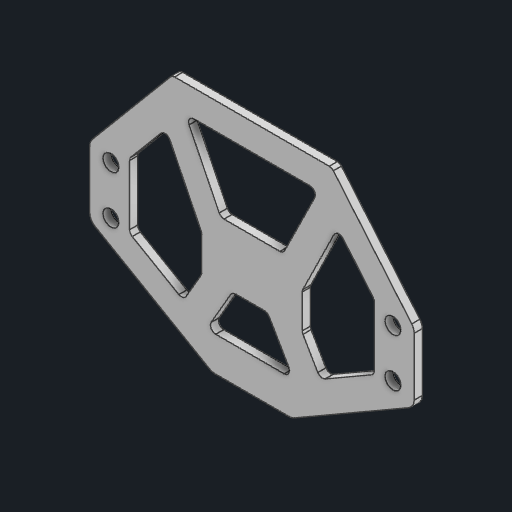
# Autodesk Inventor part: JawMount
Saved by Autodesk Inventor 2025.2 (Build 292293000, 293)
## iProperties
Created: 2024-12-21
Part Number: JawMount
Material: Generic
Document SubType Name: Sheet Metal
Designer: valer
Density: 1 g/cm^3
Sheet Metal Rule: Default
Appearance: Default
Author: valer
Autodesk Inventor part; units mm, degrees
ref_plane "YZ Plane" through (0, 0, 0) normal (1, 0, 0) x (0, 1, 0)
ref_plane "XZ Plane" through (0, 0, 0) normal (0, 1, 0) x (-1, 0, 0)
ref_plane "XY Plane" through (0, 0, 0) normal (0, 0, 1) x (1, 0, 0)
sketch "Sketch1" plane through (0, 0, 0) normal (0, 0, 1) x (1, 0, 0)
  circle A0 centre (-3.2439, -112.6362) radius 2.7 construction
  circle A1 centre (-3.2439, -130.6362) radius 2.7 construction
  line L0 (49.7615, -342.4426) -> (49.7615, 314.6303) construction
  line L1 (-11.2439, -109.7245) -> (-11.2439, -135.255)
  line L2 (-11.2439, -109.7245) -> (19.7615, -72.7737)
  line L3 (19.7615, -72.7737) -> (49.7615, -72.7737)
  circle A2 centre (-3.2439, -112.6362) radius 3
  circle A3 centre (-3.2439, -130.6362) radius 3
  line L4 (-11.2439, -135.255) -> (34.7615, -161.8162)
  line L5 (34.7615, -161.8162) -> (49.7615, -161.8162)
  line L6 (110.7669, -109.7245) -> (110.7669, -135.255)
  line L7 (110.7669, -109.7245) -> (79.7615, -72.7737)
  line L8 (79.7615, -72.7737) -> (49.7615, -72.7737)
  circle A4 centre (102.7669, -112.6362) radius 3
  circle A5 centre (102.7669, -130.6362) radius 3
  line L9 (110.7669, -135.255) -> (64.7615, -161.8162)
  line L10 (64.7615, -161.8162) -> (49.7615, -161.8162)
  point P0 (0, 0)
  dimension "d0" = 6
  dimension "d1" = 6
  dimension "d8" = 8
  dimension "d16" = 30
  dimension "d17" = 15
  dimension "d18" = 60
  dimension "d19" = 40
  dimension "d20" = 8
  dimension "d21" = 8
  measures "d0" diameter of A2
  measures "d1" diameter of A3
  measures "d8" distance from line of L2 A0.centre
  measures "d16" distance of L2.end L3.end
  measures "d17" distance of L4.end L5.end
  measures "d18" angle of L0 L4
  measures "d19" angle of L0 L2
  measures "d20" distance from line of A1.centre L1
  measures "d21" distance from line of L4 A3.centre
extrude "Plate1" add sketch "Sketch1" along normal blind 3.048
fillet "Fillet1" radius 4 6 edges at (-11.2439, -135.255, 1.524) (-11.2439, -109.7245, 1.524) (110.7669, -109.7245, 1.524) (110.7669, -135.255, 1.524) (64.7615, -161.8162, 1.524) (34.7615, -161.8162, 1.524)
sketch "Sketch2" plane through (0, 0, 3.048) normal (0, 0, 1) x (1, 0, 0)
  arc A0 (19.774, -118.0434) -> (18.9211, -121.2485) centre (16.9316, -119.0031) ccw projected
  arc A1 (80.0915, -120.6614) -> (80.0915, -117.3448) centre (82.5915, -119.0031) ccw projected
  arc A2 (47.082, -94.8758) -> (52.441, -94.8758) centre (49.7615, -96.225) ccw projected
  line L0 (3.7561, -107.7275) -> (3.7561, -132.1292)
  line L1 (3.7561, -107.7275) -> (17.5274, -91.3156)
  line L2 (17.5274, -91.3156) -> (30.8475, -118.3156)
  line L3 (30.8475, -118.3156) -> (30.8475, -131.9856)
  line L4 (30.8475, -131.9856) -> (24.0125, -143.8242)
  line L5 (24.0125, -143.8242) -> (3.7561, -132.1292)
  line L6 (24.6949, -82.7737) -> (38.0151, -109.7737)
  line L7 (38.0151, -109.7737) -> (61.508, -109.7737)
  line L8 (19.7615, -72.7737) -> (79.7615, -72.7737) projected
  line L9 (61.508, -109.7737) -> (74.8281, -82.7737)
  line L10 (74.8281, -82.7737) -> (24.6949, -82.7737)
  line L11 (-10.308, -108.6092) -> (19.7615, -72.7737) projected
  line L12 (33.8333, -161.2803) -> (-9.2439, -136.4097) projected
  line L13 (-11.2439, -132.9456) -> (-11.2439, -111.1803) projected
  arc A3 (63.6897, -161.8162) -> (65.6897, -161.2803) centre (63.6897, -157.8162) ccw projected
  line L14 (19.7615, -72.7737) -> (63.6897, -161.8162) construction
  line L15 (17.5274, -91.3156) -> (24.6949, -82.7737) construction
  line L16 (38.0151, -109.7737) -> (30.8475, -118.3156) construction
  line L17 (49.7615, -82.7737) -> (49.7615, -72.7737) construction
  line L18 (79.7615, -72.7737) -> (109.8311, -108.6092) projected
  line L19 (35.8333, -161.8162) -> (63.6897, -161.8162) projected
  line L20 (79.7615, -72.7737) -> (35.8333, -161.8162) construction
  line L21 (95.7669, -107.7275) -> (95.7669, -132.1292)
  line L22 (95.7669, -107.7275) -> (81.9957, -91.3156)
  line L23 (81.9957, -91.3156) -> (68.6755, -118.3156)
  line L24 (68.6755, -118.3156) -> (68.6755, -131.9856)
  line L25 (68.6755, -131.9856) -> (75.5105, -143.8242)
  line L26 (75.5105, -143.8242) -> (95.7669, -132.1292)
  line L27 (42.3946, -131.9856) -> (32.6728, -148.8242)
  line L28 (32.6728, -148.8242) -> (65.3755, -148.8242)
  line L29 (65.3755, -148.8242) -> (55.6538, -131.9856)
  line L30 (55.6538, -131.9856) -> (42.3946, -131.9856)
  line L31 (30.8475, -131.9856) -> (68.6755, -131.9856) construction
  line L32 (24.0125, -143.8242) -> (32.6728, -148.8242) construction
  line L33 (65.3755, -148.8242) -> (75.5105, -143.8242) construction
  point P0 (0, 0)
  point P1 (37.5337, -140.4049)
  dimension "d22" = 10
  dimension "d23" = 15
  dimension "d24" = 27
  dimension "d25" = 10.2071
  dimension "d26" = 10.2071
  dimension "d27" = 10.2071
  dimension "d28" = 10
  constraints: 56 end point, 9 parallel, 6 symmetric about line, 5 collinear, 4 perpendicular, 3 midpoint, 2 horizontal, 2 vertical, 1 equal length
  measures "d22" distance between parallel lines of L8 L10
  measures "d23" distance between parallel lines of L13 L0
  measures "d24" distance between parallel lines of L10 L7
  measures "d25" distance between parallel lines of L11 L1
  measures "d26" distance between parallel lines of L12 L5
  measures "d27" distance between parallel lines of L6 L2
  measures "d28" distance from line of point (37.534, -140.405) L4
extrude "Cut1" cut sketch "Sketch2" against normal blind 3.048
fillet "Fillet2" radius 2 22 edges at (19.7615, -72.7737, 1.524) (79.7615, -72.7737, 1.524) (17.5274, -91.3156, 1.524) (3.7561, -107.7275, 1.524) (3.7561, -132.1292, 1.524) (24.0125, -143.8242, 1.524) (30.8475, -131.9856, 1.524) (30.8475, -118.3156, 1.524) (74.8281, -82.7737, 1.524) (24.6949, -82.7737, 1.524) (38.0151, -109.7737, 1.524) (61.508, -109.7737, 1.524) (81.9957, -91.3156, 1.524) (68.6755, -118.3156, 1.524) (68.6755, -131.9856, 1.524) (75.5105, -143.8242, 1.524) (95.7669, -132.1292, 1.524) (95.7669, -107.7275, 1.524) (55.6538, -131.9856, 1.524) (42.3946, -131.9856, 1.524) (32.6728, -148.8242, 1.524) (65.3755, -148.8242, 1.524)
equation "\"d26\" = d25"
equation "\"d27\" = d25"
equation "\"d10\" = Thickness"
equation "\"BendRadius\" = Thickness"
equation "\"BendReliefWidth\" = Thickness"
equation "\"BendReliefDepth\" = 0.5 * Thickness"
equation "\"CornerReliefSize\" = 4 * Thickness"
equation "\"MinimumRemnant\" = 2 * Thickness"
equation "\"TransitionRadius\" = BendRadius"
equation "\"JacobiRadiusSize\" = BendRadius"
equation "\"GapSize\" = Thickness"
equation "\"Thickness\" = 3.048"
body "Solid1"
